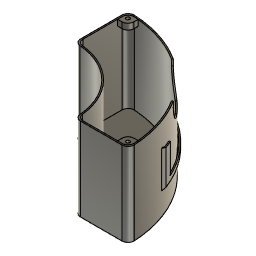
Drawer One Section v4 (Autodesk Fusion 360 design; units mm, degrees)
Autodesk Fusion 360 part; units mm, degrees
sketch "Sketch1" plane through (0, 0, 0) normal (0, 0, 1) x (1, 0, 0)
  circle A0 centre (0, 0) radius 100
  circle A1 centre (0, 0) radius 55
  line L0 (0, 0) -> (-100, 0)
  line L1 (-100, 0) -> (100, 0)
  line L2 (0, 100) -> (0, -100)
  dimension "d1" = 200
  dimension "d2" = 110
  dimension "d3" = 42.5
  constraint coincident A0.centre A1.centre
  constraint concentric A0 A1
  constraint horizontal L0
  constraint coincident A0 L1.end
  constraint parallel L0 L1
  constraint coincident A0 L2.start
  constraint coincident A0 L2.end
  constraint perpendicular L1 L2
  measures "d1" diameter of A0
  measures "d2" diameter of A1
extrude "Extrude1" add sketch "Sketch1" along normal blind 2 contours A0 A1 L1 L2 picked at (4.7438, 84.6607) makes body 1
sketch "Sketch2" plane through (0, 0, 2) normal (0, 0, 1) x (-1, 0, 0)
  line L0 (-55, 0) -> (-100, 0)
  arc A0 (-100, 0) -> (0, -100) centre (0, 0) ccw
  line L1 (0, -100) -> (0, -55)
  arc A1 (-55, 0) -> (0, -55) centre (0, 0) ccw
  circle A2 centre (0, 0) radius 56.05
  circle A3 centre (0, 0) radius 100.1
  circle A4 centre (0, 0) radius 98.9
  line L2 (0, -100) -> (0, -55)
  line L3 (-55, 0) -> (-100, 0)
  line L4 (-56.0372, -1.2) -> (-98.8927, -1.2)
  line L5 (-1.2, -98.8927) -> (-1.2, -56.0372)
  circle A5 centre (0, 0) radius 55
  dimension "d6" = 112.1
  dimension "d7" = 197.8
  dimension "d8" = 1.2
  dimension "d10" = 1.2
  dimension "d13" = 1.2
  constraint concentric A0 A2
  constraint concentric A2 A4
  constraint coincident A0.end L1.start
  constraint coincident L1.end A1.end
  constraint coincident L0.start A1.start
  constraint coincident L0.end A0.start
  constraint coincident A2 L4.start
  constraint coincident A4 L4.end
  constraint parallel L3 L4
  constraint coincident A4 L5.start
  constraint coincident A2 L5.end
  constraint parallel L2 L5
  constraint concentric A4 A5
  constraint coincident L1.end A5
  measures "d6" diameter of A2
  measures "d7" diameter of A4
  measures "d8" distance of L3 L4
  measures "d10" distance of L2 L5
  measures "d13" distance of A3 A4
extrude "Extrude2" add sketch "Sketch2" along normal blind 68 contours L0 L1 A1 A2 L2 L3 A5 | L0 A2 A4 L3 L4 | L0 A0 L1 A4 L2 L3 | L1 A2 A4 L2 L5 bodies 1
fillet "Fillet1" radius 5 4 edges at (1.2, 98.8927, 36) (56.0372, 1.2, 36) (1.2, 56.0372, 36) (98.8927, 1.2, 36) on bodies 1
fillet "Fillet1" radius 5 4 edges at (0, 100, 35) (0, 55, 35) (55, 0, 35) (100, 0, 35) on bodies 1
sketch "Sketch3" plane through (0, 0, 70) normal (0, 0, 1) x (-1, 0, 0)
  arc A0 (-94.8683, 0) -> (-99.8614, -5.2632) centre (-94.8683, -5) ccw
  arc A1 (-99.8614, -5.2632) -> (-5.2632, -99.8614) centre (0, 0) ccw
  arc A2 (-5.2632, -99.8614) -> (0, -94.8683) centre (-5, -94.8683) ccw
  line L0 (0, -94.8683) -> (0, -59.7913)
  arc A3 (0, -59.7913) -> (-4.5833, -54.8087) centre (-5, -59.7913) ccw
  arc A4 (-54.8087, -4.5833) -> (-4.5833, -54.8087) centre (0, 0) ccw
  arc A5 (-54.8087, -4.5833) -> (-59.7913, 0) centre (-59.7913, -5) ccw
  line L1 (-59.7913, 0) -> (-94.8683, 0)
  arc A6 (-98.6842, -6.5301) -> (-6.5301, -98.6842) centre (0, 0) ccw
  arc A7 (-93.6951, -1.2) -> (-98.6842, -6.5301) centre (-93.6951, -6.2) ccw
  line L2 (-93.6951, -1.2) -> (-60.7344, -1.2)
  arc A8 (-55.7602, -5.6922) -> (-60.7344, -1.2) centre (-60.7344, -6.2) ccw
  arc A9 (-55.7602, -5.6922) -> (-5.6922, -55.7602) centre (0, 0) ccw
  arc A10 (-1.2, -60.7344) -> (-5.6922, -55.7602) centre (-6.2, -60.7344) ccw
  line L3 (-1.2, -60.7344) -> (-1.2, -93.6951)
  arc A11 (-6.5301, -98.6842) -> (-1.2, -93.6951) centre (-6.2, -93.6951) ccw
  circle A12 centre (-5, -94.8683) radius 5
  line L4 (-5, -94.8683) -> (0, -94.8683)
  line L5 (0, -94.8683) -> (0, -89.8683)
  line L6 (0, -89.8683) -> (-5, -89.8683)
  line L7 (-5, -89.8683) -> (-5, -94.8683)
  line L8 (-10, -94.8683) -> (-10, -98.3931)
  line L9 (-10, -98.3931) -> (-8.3902, -98.5435)
  line L10 (-10, -98.3931) -> (-10, -99.4987)
  line L11 (-5.2632, -99.8614) -> (-10, -99.4987)
  line L12 (0, 0) -> (-87.3962, -87.3962)
  circle A13 centre (-94.8683, -5) radius 5
  line L13 (-89.8683, -5) -> (-94.8683, -5)
  line L14 (-94.8683, 0) -> (-59.7913, 0)
  arc A14 (-94.8683, 0) -> (-99.8614, -5.2632) centre (-94.8683, -5) ccw
  arc A15 (-98.6842, -6.5301) -> (-6.5301, -98.6842) centre (0, 0) ccw
  line L15 (-94.8683, -5) -> (-94.8683, 0)
  line L16 (-60.7344, -1.2) -> (-93.6951, -1.2)
  arc A16 (-55.7602, -5.6922) -> (-60.7344, -1.2) centre (-60.7344, -6.2) ccw
  arc A17 (-54.8087, -4.5833) -> (-59.7913, 0) centre (-59.7913, -5) ccw
  arc A18 (-93.6951, -1.2) -> (-98.6842, -6.5301) centre (-93.6951, -6.2) ccw
  arc A19 (-99.8614, -5.2632) -> (-5.2632, -99.8614) centre (0, 0) ccw
  line L17 (-60.7344, -1.2) -> (-93.6951, -1.2)
  line L18 (-94.8683, 0) -> (-59.7913, 0)
  line L19 (-89.8683, -5) -> (-94.8683, -5)
  line L20 (-94.8683, -5) -> (-94.8683, 0)
  arc A20 (-93.6951, -1.2) -> (-98.6842, -6.5301) centre (-93.6951, -6.2) ccw
  line L21 (-89.8683, 0) -> (-89.8683, -5)
  line L22 (-98.3931, -10) -> (-98.5435, -8.3902)
  arc A21 (-98.6842, -6.5301) -> (-6.5301, -98.6842) centre (0, 0) ccw
  arc A22 (-99.8614, -5.2632) -> (-5.2632, -99.8614) centre (0, 0) ccw
  line L23 (-98.3931, -10) -> (-99.4987, -10)
  circle A23 centre (-94.8683, -5) radius 5
  line L24 (-99.8614, -5.2632) -> (-99.4987, -10)
  arc A24 (-99.8614, -5.2632) -> (-5.2632, -99.8614) centre (0, 0) ccw
  line L25 (-94.8683, 0) -> (-89.8683, 0)
  arc A25 (-94.8683, 0) -> (-99.8614, -5.2632) centre (-94.8683, -5) ccw
  arc A26 (-98.6842, -6.5301) -> (-6.5301, -98.6842) centre (0, 0) ccw
  line L26 (-94.8683, -10) -> (-98.3931, -10)
  point P0 (-94.8683, -10)
  dimension "d16" = 5
  dimension "d20" = 45
  constraint concentric A2 A12
  constraint horizontal L4
  constraint vertical L5
  constraint horizontal L6
  constraint vertical L7
  constraint coincident A2.centre A12.centre
  constraint coincident A12 L8.start
  constraint coincident A6 L8.end
  constraint tangent A12 L8
  constraint vertical L8
  constraint coincident A12 L9.end
  constraint coincident A6 L9.end
  constraint coincident A1 L10.end
  constraint parallel L8 L10
  constraint coincident A1.end A2.start
  constraint coincident A1.centre A4.centre
  constraint symmetric A0.end L12 A1.end
  constraint symmetric A1.end L12 A0.end
  constraint symmetric A1 L12 A19
  constraint symmetric A2.end L12 A0.start
  constraint symmetric A2 L12 A14
  constraint symmetric L0.end L12 A5.end
  constraint symmetric A3.end L12 A4.start
  constraint symmetric A3 L12 A17
  constraint symmetric A6.start L12 A6.end
  constraint symmetric A6.end L12 A6.start
  constraint symmetric A6 L12 A15
  constraint symmetric A9.end L12 A8.start
  constraint symmetric A10.start L12 L2.end
  constraint symmetric A10 L12 A16
  constraint symmetric L3.end L12 A7.start
  constraint symmetric A11 L12 A18
  constraint symmetric A12 L12 A13
  constraint symmetric A2.centre L12 A0.centre
  constraint symmetric L6.end L12 L13.start
  constraint symmetric L8.start L12 P0
  constraint symmetric A1 L12 A22
  constraint symmetric A2 L12 A25
  constraint symmetric A6 L12 A21
  constraint symmetric A11 L12 A20
  constraint symmetric A12 L12 A23
  constraint symmetric L5.end L12 L21.start
  constraint symmetric L8.end L12 L22.start
  constraint symmetric L9.end L12 L22.end
  constraint symmetric L10.end L12 L23.end
  constraint symmetric L12 A0.end A1.end
  constraint symmetric L12 A6.end A6.start
  constraint symmetric L12 A6.start A6.end
  constraint symmetric L12 A15 A26
  constraint symmetric L12 A1.end A0.end
  constraint symmetric L12 A19 A24
  measures "d16" distance of A2.centre L6.end
  measures "d20" angle of L1 L12
extrude "Extrude3" add sketch "Sketch3" against normal blind 5 separate body contours A7 L2 A13 L13 L15 L16 A18 L17 L19 L20 A20 A23 | L2 A13 L16 L17 L21 A23 | A6 A7 A13 L13 A15 L15 A18 L19 L20 A20 A21 A23 A26 | A13 L22 A23 L26 | A12 L8 L9 | A6 A11 A12 L4 L7 A15 A21 A26 | L3 A12 L6 | L3 A11 A12 L4 L7 makes body 2 at (2.4667, 91.1439, 65) makes body 3 at (91.1439, 2.4667, 70)
sketch "Sketch4" plane through (0, 0, 70) normal (0, 0, 1) x (-1, 0, 0)
  line L0 (-1.2, -89.8683) -> (-5, -89.8683)
  arc A0 (-5, -89.8683) -> (-10, -94.8683) centre (-5, -94.8683) ccw
  line L1 (-10, -94.8683) -> (-10, -98.3931)
  line L2 (-10, -98.3931) -> (-8.3902, -98.5435)
  arc A1 (-8.3902, -98.5435) -> (-6.5301, -98.6842) centre (0, 0) ccw
  arc A2 (-6.5301, -98.6842) -> (-1.2, -93.6951) centre (-6.2, -93.6951) ccw
  line L3 (-1.2, -93.6951) -> (-1.2, -89.8683)
  circle A3 centre (-5, -94.8683) radius 1.5
  dimension "d21" = 5
  dimension "d22" = 3
  constraint concentric A0 A3
  measures "d21" radius of A0
  measures "d22" diameter of A3
extrude "Extrude4" cut sketch "Sketch4" against normal blind 10 contours A3 bodies 2
sketch "Sketch5" plane through (0, 0, 65) normal (0, 0, -1) x (1, 0, 0)
  circle A0 centre (5, -94.8683) radius 1.5
  line L0 (5, -89.8683) -> (1.2, -89.8683)
  line L1 (1.2, -89.8683) -> (1.2, -93.6951)
  arc A1 (1.2, -93.6951) -> (6.5301, -98.6842) centre (6.2, -93.6951) ccw
  arc A2 (6.5301, -98.6842) -> (8.3902, -98.5435) centre (0, 0) ccw
  line L2 (8.3902, -98.5435) -> (10, -98.3931)
  line L3 (10, -98.3931) -> (10, -94.8683)
  arc A3 (10, -94.8683) -> (5, -89.8683) centre (5, -94.8683) ccw
  circle A4 centre (5, -94.8683) radius 3
  dimension "d25" = 6
  constraint concentric A0 A4
  measures "d25" diameter of A4
extrude "Extrude5" cut sketch "Sketch5" against normal blind 3 contours A4 bodies 2
sketch "Sketch6" plane through (0, 0, 70) normal (0, 0, 1) x (-1, 0, 0)
  line L0 (-89.8683, -1.2) -> (-93.6951, -1.2)
  arc A0 (-93.6951, -1.2) -> (-98.6842, -6.5301) centre (-93.6951, -6.2) ccw
  arc A1 (-98.6842, -6.5301) -> (-98.5435, -8.3902) centre (0, 0) ccw
  line L1 (-98.5435, -8.3902) -> (-98.3931, -10)
  line L2 (-98.3931, -10) -> (-94.8683, -10)
  arc A2 (-94.8683, -10) -> (-89.8683, -5) centre (-94.8683, -5) ccw
  line L3 (-89.8683, -5) -> (-89.8683, -1.2)
  circle A3 centre (-94.8683, -5) radius 1.5
  dimension "d28" = 5
  dimension "d29" = 3
  constraint concentric A2 A3
  measures "d28" radius of A2
  measures "d29" diameter of A3
extrude "Extrude6" cut sketch "Sketch6" against normal blind 10 contours A3 bodies 3
sketch "Sketch7" plane through (0, 0, 65) normal (0, 0, -1) x (1, 0, 0)
  circle A0 centre (94.8683, -5) radius 1.5
  line L0 (93.6951, -1.2) -> (89.8683, -1.2)
  line L1 (89.8683, -1.2) -> (89.8683, -5)
  arc A1 (89.8683, -5) -> (94.8683, -10) centre (94.8683, -5) ccw
  line L2 (94.8683, -10) -> (98.3931, -10)
  line L3 (98.3931, -10) -> (98.5435, -8.3902)
  arc A2 (98.5435, -8.3902) -> (98.6842, -6.5301) centre (0, 0) ccw
  arc A3 (98.6842, -6.5301) -> (93.6951, -1.2) centre (93.6951, -6.2) ccw
  circle A4 centre (94.8683, -5) radius 3
  dimension "d32" = 6
  constraint concentric A0 A4
  measures "d32" diameter of A4
extrude "Extrude7" cut sketch "Sketch7" against normal blind 3 contours A4 bodies 3
sketch "Sketch8" plane through (0, 0, 70) normal (0, 0, 1) x (-1, 0, 0)
  line L0 (-93.6951, -1.2) -> (-60.7344, -1.2)
  arc A0 (-55.7602, -5.6922) -> (-60.7344, -1.2) centre (-60.7344, -6.2) ccw
  arc A1 (-55.7602, -5.6922) -> (-5.6922, -55.7602) centre (0, 0) ccw
  arc A2 (-1.2, -60.7344) -> (-5.6922, -55.7602) centre (-6.2, -60.7344) ccw
  line L1 (-1.2, -60.7344) -> (-1.2, -93.6951)
  arc A3 (-6.5301, -98.6842) -> (-1.2, -93.6951) centre (-6.2, -93.6951) ccw
  arc A4 (-98.6842, -6.5301) -> (-6.5301, -98.6842) centre (0, 0) ccw
  arc A5 (-93.6951, -1.2) -> (-98.6842, -6.5301) centre (-93.6951, -6.2) ccw
  arc A6 (-94.8683, 0) -> (-99.8614, -5.2632) centre (-94.8683, -5) ccw
  arc A7 (-99.8614, -5.2632) -> (-5.2632, -99.8614) centre (0, 0) ccw
  arc A8 (-5.2632, -99.8614) -> (0, -94.8683) centre (-5, -94.8683) ccw
  line L2 (0, -94.8683) -> (0, -59.7913)
  arc A9 (0, -59.7913) -> (-4.5833, -54.8087) centre (-5, -59.7913) ccw
  arc A10 (-54.8087, -4.5833) -> (-4.5833, -54.8087) centre (0, 0) ccw
  arc A11 (-54.8087, -4.5833) -> (-59.7913, 0) centre (-59.7913, -5) ccw
  line L3 (-59.7913, 0) -> (-94.8683, 0)
  circle A12 centre (0, 0) radius 102
  line L4 (0, 0) -> (-34.8861, -95.8486)
  line L5 (0, 0) -> (-95.8486, -34.8861)
  circle A13 centre (0, 0) radius 101
  circle A14 centre (0, 0) radius 100
  circle A15 centre (0, 0) radius 100
  line L6 (0, 0) -> (-36.5535, -95.2252)
  line L7 (0, 0) -> (-95.2252, -36.5535)
  dimension "d35" = 204
  dimension "d36" = 50
  dimension "d37" = 20
  dimension "d38" = 20
  dimension "d41" = 1
  dimension "d42" = 1
  dimension "d51" = 1
  constraint concentric A1 A12
  constraint coincident A1.centre A4.centre
  constraint coincident A12 L4.end
  constraint coincident A12 L5.end
  constraint concentric A13 A14
  constraint concentric A14 A15
  constraint coincident A12 L6.end
  constraint coincident A12 L7.end
  measures "d35" diameter of A12
  measures "d36" angle of L4 L5
  measures "d37" angle of L3 L5
  measures "d38" angle of L2 L4
  measures "d41" angle of L4 L6
  measures "d42" angle of L5 L7
  measures "d51" distance of A13 A14
extrude "Extrude8" add sketch "Sketch8" against normal blind 50 contours A7 L5 A13 A14 A15 L7 | A12 L5 A13 L7 | A7 L4 A13 A14 A15 L6 | A12 A13 L6 L7 | A12 L4 A13 L6 bodies 1
sketch "Sketch9" plane through (0, 0, 70) normal (0, 0, 1) x (-1, 0, 0)
  arc A0 (-34.202, -93.9693) -> (-5.2632, -99.8614) centre (0, 0) ccw
  arc A1 (-5.2632, -99.8614) -> (0, -94.8683) centre (-5, -94.8683) ccw
  line L0 (0, -94.8683) -> (0, -59.7913)
  arc A2 (0, -59.7913) -> (-4.5833, -54.8087) centre (-5, -59.7913) ccw
  arc A3 (-54.8087, -4.5833) -> (-4.5833, -54.8087) centre (0, 0) ccw
  arc A4 (-54.8087, -4.5833) -> (-59.7913, 0) centre (-59.7913, -5) ccw
  line L1 (-59.7913, 0) -> (-94.8683, 0)
  arc A5 (-94.8683, 0) -> (-99.8614, -5.2632) centre (-94.8683, -5) ccw
  arc A6 (-99.8614, -5.2632) -> (-93.9693, -34.202) centre (0, 0) ccw
  line L2 (-93.9693, -34.202) -> (-95.8486, -34.8861)
  arc A7 (-95.8486, -34.8861) -> (-34.8861, -95.8486) centre (0, 0) ccw
  line L3 (-34.8861, -95.8486) -> (-34.202, -93.9693)
  line L4 (-93.6951, -1.2) -> (-60.7344, -1.2)
  arc A8 (-55.7602, -5.6922) -> (-60.7344, -1.2) centre (-60.7344, -6.2) ccw
  arc A9 (-55.7602, -5.6922) -> (-5.6922, -55.7602) centre (0, 0) ccw
  arc A10 (-1.2, -60.7344) -> (-5.6922, -55.7602) centre (-6.2, -60.7344) ccw
  line L5 (-1.2, -60.7344) -> (-1.2, -93.6951)
  arc A11 (-6.5301, -98.6842) -> (-1.2, -93.6951) centre (-6.2, -93.6951) ccw
  arc A12 (-98.6842, -6.5301) -> (-6.5301, -98.6842) centre (0, 0) ccw
  arc A13 (-93.6951, -1.2) -> (-98.6842, -6.5301) centre (-93.6951, -6.2) ccw
  line L6 (-35.8368, -93.358) -> (-36.1952, -94.2916)
  arc A14 (-94.2916, -36.1952) -> (-36.1952, -94.2916) centre (0, 0) ccw
  line L7 (-94.2916, -36.1952) -> (-93.358, -35.8368)
  arc A15 (-93.358, -35.8368) -> (-35.8368, -93.358) centre (0, 0) ccw
  circle A16 centre (0, 0) radius 103
  circle A17 centre (0, 0) radius 100
  constraint coincident A0.centre A3.centre
  constraint concentric A0 A17
extrude "Extrude9" cut sketch "Sketch9" against normal blind 20 contours L2 A7 L3 L6 A14 L7 A17 | L6 A14 L7 A15 A17 | A16 bodies 1
sketch "Sketch10" plane through (0, 0, 20) normal (0, 0, -1) x (1, 0, 0)
  line L0 (95.8486, -34.8861) -> (93.9693, -34.202)
  arc A0 (93.358, -35.8368) -> (93.9693, -34.202) centre (0, 0) ccw
  line L1 (93.358, -35.8368) -> (94.2916, -36.1952)
  arc A1 (36.1952, -94.2916) -> (94.2916, -36.1952) centre (0, 0) ccw
  line L2 (36.1952, -94.2916) -> (35.8368, -93.358)
  arc A2 (34.202, -93.9693) -> (35.8368, -93.358) centre (0, 0) ccw
  line L3 (34.202, -93.9693) -> (34.8861, -95.8486)
  arc A3 (34.8861, -95.8486) -> (95.8486, -34.8861) centre (0, 0) ccw
  circle A4 centre (0, 0) radius 103
  circle A5 centre (0, 0) radius 100
  line L4 (34.8861, -95.8486) -> (0, 0)
  line L5 (0, 0) -> (95.8486, -34.8861)
  dimension "d47" = 200
  constraint concentric A0 A4
  constraint concentric A0 A5
  constraint coincident L3.end A3.start
  constraint coincident A0.centre A1.centre
  constraint coincident L0.start A3.end
  measures "d47" diameter of A5
extrude "Extrude10" add sketch "Sketch10" along normal blind 1 contours L0 A0 L1 A1 L2 A2 L3 A3 A5 L4 L5 | L1 A1 L2 A5 bodies 1
chamfer "Chamfer1" distance 2 angle 45 3 edges at (95.8486, 34.8861, 34.5) (72.1249, 72.1249, 19) (34.8861, 95.8486, 34.5) on bodies 1
sketch "Sketch11" plane through (0, 0, 70) normal (0, 0, 1) x (-1, 0, 0)
  arc A0 (-99.8614, -5.2632) -> (-5.2632, -99.8614) centre (0, 0) ccw
  arc A1 (-5.2632, -99.8614) -> (0, -94.8683) centre (-5, -94.8683) ccw
  line L0 (0, -94.8683) -> (0, -59.7913)
  arc A2 (0, -59.7913) -> (-4.5833, -54.8087) centre (-5, -59.7913) ccw
  arc A3 (-54.8087, -4.5833) -> (-4.5833, -54.8087) centre (0, 0) ccw
  arc A4 (-54.8087, -4.5833) -> (-59.7913, 0) centre (-59.7913, -5) ccw
  line L1 (-59.7913, 0) -> (-94.8683, 0)
  arc A5 (-94.8683, 0) -> (-99.8614, -5.2632) centre (-94.8683, -5) ccw
  line L2 (-93.6951, -1.2) -> (-60.7344, -1.2)
  arc A6 (-55.7602, -5.6922) -> (-60.7344, -1.2) centre (-60.7344, -6.2) ccw
  arc A7 (-55.7602, -5.6922) -> (-5.6922, -55.7602) centre (0, 0) ccw
  arc A8 (-1.2, -60.7344) -> (-5.6922, -55.7602) centre (-6.2, -60.7344) ccw
  line L3 (-1.2, -60.7344) -> (-1.2, -93.6951)
  arc A9 (-6.5301, -98.6842) -> (-1.2, -93.6951) centre (-6.2, -93.6951) ccw
  arc A10 (-98.6842, -6.5301) -> (-6.5301, -98.6842) centre (0, 0) ccw
  arc A11 (-93.6951, -1.2) -> (-98.6842, -6.5301) centre (-93.6951, -6.2) ccw
  circle A12 centre (0, 0) radius 102
  circle A13 centre (0, 0) radius 100
  line L4 (0, 0) -> (-43.1071, -92.4434)
  line L5 (0, 0) -> (-92.4434, -43.1071)
  dimension "d52" = 40
  dimension "d53" = 25
  dimension "d54" = 22.5
  dimension "d57" = 204
  constraint concentric A0 A12
  constraint coincident A0.centre A3.centre
  constraint coincident A12 L4.end
  constraint coincident A12 L5.end
  measures "d52" angle of L4 L5
  measures "d53" angle of L1 L5
  measures "d57" diameter of A12
extrude "Extrude11" cut sketch "Sketch11" against normal blind 45 contours A0 A12 A13 L4 L5 picked at (-79.3319, -62.6924) bodies 1
sketch "Sketch12" plane through (0, 0, 70) normal (0, 0, 1) x (-1, 0, 0)
  arc A0 (-99.8614, -5.2632) -> (-5.2632, -99.8614) centre (0, 0) ccw
  arc A1 (-5.2632, -99.8614) -> (0, -94.8683) centre (-5, -94.8683) ccw
  line L0 (0, -94.8683) -> (0, -59.7913)
  arc A2 (0, -59.7913) -> (-4.5833, -54.8087) centre (-5, -59.7913) ccw
  arc A3 (-54.8087, -4.5833) -> (-4.5833, -54.8087) centre (0, 0) ccw
  arc A4 (-54.8087, -4.5833) -> (-59.7913, 0) centre (-59.7913, -5) ccw
  line L1 (-59.7913, 0) -> (-94.8683, 0)
  arc A5 (-94.8683, 0) -> (-99.8614, -5.2632) centre (-94.8683, -5) ccw
  line L2 (-93.6951, -1.2) -> (-60.7344, -1.2)
  arc A6 (-55.7602, -5.6922) -> (-60.7344, -1.2) centre (-60.7344, -6.2) ccw
  arc A7 (-55.7602, -5.6922) -> (-5.6922, -55.7602) centre (0, 0) ccw
  arc A8 (-1.2, -60.7344) -> (-5.6922, -55.7602) centre (-6.2, -60.7344) ccw
  line L3 (-1.2, -60.7344) -> (-1.2, -93.6951)
  arc A9 (-6.5301, -98.6842) -> (-1.2, -93.6951) centre (-6.2, -93.6951) ccw
  arc A10 (-98.6842, -6.5301) -> (-6.5301, -98.6842) centre (0, 0) ccw
  arc A11 (-93.6951, -1.2) -> (-98.6842, -6.5301) centre (-93.6951, -6.2) ccw
  circle A12 centre (0, 0) radius 100
  circle A13 centre (0, 0) radius 98.9
  line L4 (0, 0) -> (-53.73, -84.3391)
  line L5 (0, 0) -> (-84.3391, -53.73)
  dimension "d58" = 25
  dimension "d59" = 32.5
  constraint coincident A0.centre A3.centre
  constraint concentric A0 A13
  constraint coincident A12 L4.end
  constraint coincident A0 L4.end
  constraint coincident A12 L5.end
  measures "d58" angle of L4 L5
  measures "d59" angle of L1 L5
extrude "Extrude12" cut sketch "Sketch12" against normal blind 20 contours A0 A10 A12 A13 L4 L5 bodies 1
sketch "Sketch13" plane through (0, 0, 70) normal (0, 0, 1) x (-1, 0, 0)
  line L0 (-84.3391, -53.73) -> (-83.4114, -53.1389)
  arc A0 (-98.6842, -6.5301) -> (-83.4114, -53.1389) centre (0, 0) ccw
  arc A1 (-93.6951, -1.2) -> (-98.6842, -6.5301) centre (-93.6951, -6.2) ccw
  line L1 (-93.6951, -1.2) -> (-60.7344, -1.2)
  arc A2 (-55.7602, -5.6922) -> (-60.7344, -1.2) centre (-60.7344, -6.2) ccw
  arc A3 (-55.7602, -5.6922) -> (-5.6922, -55.7602) centre (0, 0) ccw
  arc A4 (-1.2, -60.7344) -> (-5.6922, -55.7602) centre (-6.2, -60.7344) ccw
  line L2 (-1.2, -60.7344) -> (-1.2, -93.6951)
  arc A5 (-6.5301, -98.6842) -> (-1.2, -93.6951) centre (-6.2, -93.6951) ccw
  arc A6 (-53.1389, -83.4114) -> (-6.5301, -98.6842) centre (0, 0) ccw
  line L3 (-53.1389, -83.4114) -> (-53.73, -84.3391)
  arc A7 (-53.73, -84.3391) -> (-5.2632, -99.8614) centre (0, 0) ccw
  arc A8 (-5.2632, -99.8614) -> (0, -94.8683) centre (-5, -94.8683) ccw
  line L4 (0, -94.8683) -> (0, -59.7913)
  arc A9 (0, -59.7913) -> (-4.5833, -54.8087) centre (-5, -59.7913) ccw
  arc A10 (-54.8087, -4.5833) -> (-4.5833, -54.8087) centre (0, 0) ccw
  arc A11 (-54.8087, -4.5833) -> (-59.7913, 0) centre (-59.7913, -5) ccw
  line L5 (-59.7913, 0) -> (-94.8683, 0)
  arc A12 (-94.8683, 0) -> (-99.8614, -5.2632) centre (-94.8683, -5) ccw
  arc A13 (-99.8614, -5.2632) -> (-84.3391, -53.73) centre (0, 0) ccw
  circle A14 centre (0, 0) radius 100
  circle A15 centre (0, 0) radius 98.9
  line L6 (0, 0) -> (-53.73, -84.3391)
  line L7 (0, 0) -> (-84.3391, -53.73)
  constraint coincident A0.centre A3.centre
  constraint concentric A14 A15
  constraint coincident L3.end A7.start
  constraint coincident L0.start A13.end
fillet "Fillet2" radius 15 2 edges at (53.4344, 83.8753, 50) (83.8753, 53.4344, 50) on bodies 1
equation "d59 = ( ( 90 - 25 ) / 2 ) * 1 deg"
